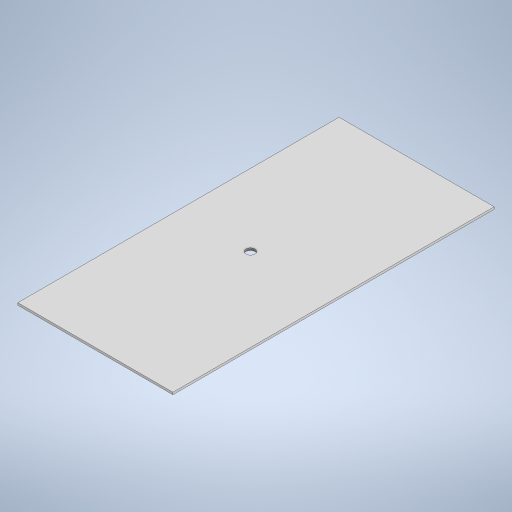
# Autodesk Inventor part: Стена 16 мм отверстие
Saved by Autodesk Inventor 2023 (Build 270158000, 158)
## iProperties
Created: 2022-05-01
Part Number: Стена 16 мм отверстие
Material: Типовые
Document SubType Name: Modeling
Designer: User
Density: 1 g/cm^3
Appearance: По умолчанию
Author: User
Autodesk Inventor part; units mm, degrees
ref_plane "YZ Plane" through (0, 0, 0) normal (1, 0, 0) x (0, 1, 0)
ref_plane "XZ Plane" through (0, 0, 0) normal (0, 1, 0) x (-1, 0, 0)
ref_plane "XY Plane" through (0, 0, 0) normal (0, 0, 1) x (1, 0, 0)
sketch "Эскиз1" plane through (0, 0, 0) normal (0, 1, 0) x (-1, 0, 0)
  line L0 (0, 0) -> (280, 0)
  line L1 (280, 0) -> (280, -580)
  line L2 (280, -580) -> (0, -580)
  line L3 (0, -580) -> (0, 0)
  circle A0 centre (150, -290) radius 8
  line L4 (150, -290) -> (0, -290)
  dimension "d0" = 280
  dimension "d1" = 580
  dimension "d2" = 16
  dimension "d3" = 150
  constraints: 10 end point, 2 parallel, 1 centre point, 1 horizontal, 1 midpoint, 1 perpendicular
  measures "d0" distance of L1.end L2.end
  measures "d1" distance of L0.end L1.end
  measures "d2" diameter of A0
  measures "d3" distance of L4.start L4.end
extrude "Выдавливание1" add sketch "Эскиз1" along normal blind 4
